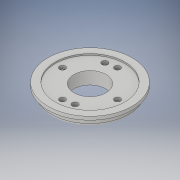
# Autodesk Inventor part: 2016.06.09 Mount Adapter
Saved by Autodesk Inventor 2017 (Build 210142000, 142)
## iProperties
Created: 2016-06-09
Part Number: 2016.06.09 Mount Adapter
Material: Generic
Document SubType Name: Modeling
Designer: Darien Morrow
Density: 1 g/cm^3
Appearance: Default
Author: Darien Morrow
Autodesk Inventor part; units mm, degrees
ref_plane "YZ Plane" through (0, 0, 0) normal (1, 0, 0) x (0, 1, 0)
ref_plane "XZ Plane" through (0, 0, 0) normal (0, 1, 0) x (-1, 0, 0)
ref_plane "XY Plane" through (0, 0, 0) normal (0, 0, 1) x (1, 0, 0)
sketch "Sketch1" plane through (0, 0, 0) normal (0, 0, 1) x (1, 0, 0)
  line L0 (23.85, 0) -> (46.0756, 0)
  line L1 (46.0756, 0) -> (46.0756, 12.7)
  line L2 (46.0756, 12.7) -> (0, 12.7)
  line L3 (0, 12.7) -> (0, 0)
  line L4 (17.5514, 12.7) -> (17.5514, -2.5)
  line L5 (46.0756, 8.9662) -> (42.3672, 8.9662)
  line L6 (42.3672, 7.747) -> (42.3672, 0)
  line L7 (46.0756, 7.747) -> (42.3672, 7.747)
  line L8 (46.0756, 8.9662) -> (42.3672, 7.747)
  line L9 (0, 11.1252) -> (0, 12.7)
  line L10 (17.5514, 0) -> (23.85, 0)
  line L11 (23.85, 0) -> (23.85, -2.5)
  line L12 (23.85, -2.5) -> (0, -2.5)
  line L13 (0, -2.5) -> (0, 0)
  dimension "d0" = 46.0756
  dimension "d1" = 12.7
  dimension "d2" = 17.5514
  dimension "d3" = 3.7338
  dimension "d4" = 42.3672
  dimension "d6" = 4.953
  dimension "d14" = 23.85
  dimension "d15" = 2.5
  constraints: 28 end point, 7 point on line, 6 perpendicular, 4 parallel, 2 horizontal
  measures "d0" distance of L2.end L1.end
  measures "d1" distance of L2.end L3.end
  measures "d2" distance between parallel lines of L3 L4
  measures "d3" distance between parallel lines of L5 L2
  measures "d4" distance between parallel lines of L3 L6
  measures "d6" distance between parallel lines of L7 L2
  measures "d14" distance between parallel lines of L11 L13
  measures "d15" distance of L0.start L11.end
revolve "Revolution1" add sketch "Sketch1" angle 360 about axis through (0, 12.7, 0) along (0, -1, 0) contours L10 L4 L2 L1 L8 L6 L0 | L11 L12 L4 L10
sketch "Sketch2" plane through (0, 12.7, 0) normal (0, 1, 0) x (1, 0, 0)
  circle A0 centre (0, 0) radius 38.1
  dimension "d11" = 76.2
  constraints: 1 centre point, 1 coincident
  measures "d11" diameter of A0
extrude "Extrusion1" cut sketch "Sketch2" against normal blind 1.5748
sketch "Sketch4" plane through (0, 11.1252, 0) normal (0, 1, 0) x (1, 0, 0)
  circle A0 centre (0, 0) radius 30.1752
  line L0 (-11.5475, 27.8782) -> (11.5475, -27.8782)
  circle A1 centre (0, 0) radius 17.5514 projected
  line L1 (0, 0) -> (0, -30.1752)
  circle A2 centre (30.1752, 0) radius 3.2512 projected
  circle A3 centre (-30.1752, 0) radius 1.7018 projected
  dimension "d25" = 60.3504
  dimension "d27" = 22.5
  constraints: 5 coincident, 4 end point, 3 point on circle, 1 centre point, 1 midpoint, 1 vertical
  measures "d25" diameter of A0
  measures "d27" angle of L0 L1
hole "Hole2" at (-11.5475, 11.1252, -27.8782) at (11.5475, 11.1252, 27.8782) at (30.1752, 11.1252, 0) at (-30.1752, 11.1252, 0) direction (0, -1, 0) diameter 3.4036 end through all counterbore diameter 6.5024 counterbore depth 3.4036 clearance for "Socket Head Cap Screw ISO 4762" size "M3" standard "ISO"
sketch "Sketch5" plane through (0, 11.1252, 0) normal (0, 1, 0) x (1, 0, 0)
  circle A0 centre (0, 0) radius 30.1752
  point P0 (0, 30.1752)
  point P1 (0, -30.1752)
  dimension "d35" = 60.3504
  constraints: 2 point on circle, 1 centre point, 1 coincident
  measures "d35" diameter of A0
hole "Hole3" at (0, 11.1252, -30.1752) at (0, 11.1252, 30.1752) direction (0, -1, 0) diameter 6.35 depth 7.62
fillet "Fillet1" radius 3.175 1 edges at (-42.3672, 0, 0)
body "Solid1"
